Autodesk Fusion 360 part; units mm, degrees
note: some values were not read from the file. Set by a fixed rule: which sketch regions a step uses.
(part 3 of 3)
sketch "Sketch5 (2)" plane through (11, 0, 0) normal (1, 0, 0) x (0, 1, 0) in component "top"
  line L0 (3, 31) -> (-3, 31)
  line L1 (-3, 31) -> (-3, 15)
  line L2 (-3, 15) -> (3, 15)
  line L3 (3, 15) -> (3, 31)
  line L4 (-2, 31.5774) -> (-3, 32.1547)
  line L5 (-3, 32.1547) -> (-4, 31.5773)
  line L6 (-4, 31.5773) -> (-4, 30.4226)
  line L7 (-4, 30.4226) -> (-3, 29.8453)
  line L8 (-3, 29.8453) -> (-2, 30.4227)
  line L9 (-2, 30.4227) -> (-2, 31.5774)
  line L10 (-2, 27.5774) -> (-3, 28.1547)
  line L11 (-3, 28.1547) -> (-4, 27.5774)
  line L12 (-4, 27.5774) -> (-4, 26.4227)
  line L13 (-4, 26.4227) -> (-3, 25.8453)
  line L14 (-3, 25.8453) -> (-2, 26.4227)
  line L15 (-2, 26.4227) -> (-2, 27.5774)
  line L16 (-2, 23.5774) -> (-3, 24.1547)
  line L17 (-3, 24.1547) -> (-4, 23.5773)
  line L18 (-4, 23.5773) -> (-4, 22.4226)
  line L19 (-4, 22.4226) -> (-3, 21.8453)
  line L20 (-3, 21.8453) -> (-2, 22.4227)
  line L21 (-2, 22.4227) -> (-2, 23.5774)
  line L22 (-2, 19.5774) -> (-3, 20.1547)
  line L23 (-3, 20.1547) -> (-4, 19.5774)
  line L24 (-4, 19.5774) -> (-4, 18.4227)
  line L25 (-4, 18.4227) -> (-3, 17.8453)
  line L26 (-3, 17.8453) -> (-2, 18.4227)
  line L27 (-2, 18.4227) -> (-2, 19.5774)
  line L28 (2, 30.4227) -> (3, 29.8453)
  line L29 (3, 29.8453) -> (4, 30.4226)
  line L30 (4, 30.4226) -> (4, 31.5773)
  line L31 (4, 31.5773) -> (3, 32.1547)
  line L32 (3, 32.1547) -> (2, 31.5774)
  line L33 (2, 31.5774) -> (2, 30.4227)
  line L34 (2, 26.4227) -> (3, 25.8453)
  line L35 (3, 25.8453) -> (4, 26.4227)
  line L36 (4, 26.4227) -> (4, 27.5774)
  line L37 (4, 27.5774) -> (3, 28.1547)
  line L38 (3, 28.1547) -> (2, 27.5774)
  line L39 (2, 27.5774) -> (2, 26.4227)
  line L40 (2, 22.4227) -> (3, 21.8453)
  line L41 (3, 21.8453) -> (4, 22.4226)
  line L42 (4, 22.4226) -> (4, 23.5773)
  line L43 (4, 23.5773) -> (3, 24.1547)
  line L44 (3, 24.1547) -> (2, 23.5774)
  line L45 (2, 23.5774) -> (2, 22.4227)
  line L46 (2, 18.4227) -> (3, 17.8453)
  line L47 (3, 17.8453) -> (4, 18.4227)
  line L48 (4, 18.4227) -> (4, 19.5774)
  line L49 (4, 19.5774) -> (3, 20.1547)
  line L50 (3, 20.1547) -> (2, 19.5774)
  line L51 (2, 19.5774) -> (2, 18.4227)
  point P0 (-3, 31)
  point P1 (-3, 27)
  point P2 (-3, 23)
  point P3 (-3, 19)
  point P4 (3, 31)
  point P5 (3, 27)
  point P6 (3, 23)
  point P7 (3, 19)
  constraint coincident P0 L0.end
  constraint coincident L1 P1
  constraint midpoint L1 P2
  constraint coincident L1 P3
  constraint coincident P4 L0.start
  constraint coincident L3 P5
  constraint midpoint L3 P6
  constraint coincident L3 P7
extrude "Extrude4'" cut sketch "Sketch5 (2)" against normal blind 100 contours L0 L3 L28 L33 | L0 L3 L29 L30 L31 L32 L33 | L0 L1 L8 L9 | L0 L1 L4 L5 L6 L7 L9 | L3 L34 L38 L39 | L3 L40 L44 L45 | L1 L10 L14 L15 | L3 L46 L50 L51 | L1 L16 L20 L21 | L1 L22 L26 L27 bodies 3 in component "top"
component "top" placed x (1, 0, 0) y (0, 1, 0) z (0, 0, 1) at (0, 0, 0)
component "base" placed x (1, 0, 0) y (0, 1, 0) z (0, 0, 1) at (0, 0, 0)
